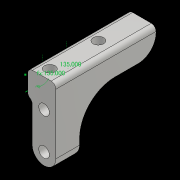
# Autodesk Inventor part: small_gpu_02
Saved by Autodesk Inventor 2018.2 (Build 222227000, 227)
## iProperties
Created: 2020-06-13
Part Number: small_gpu_02
Material: アルミニウム 6061
Document SubType Name: Modeling
Designer: gisen
Density: 2.7 g/cm^3
Appearance: アルミニウム - フラット
Author: gisen
## iProperties of the stored document small_gpu_02_3D プリント.ipt
Created: 2020-06-13
Part Number: small_gpu_02_3D プリント
Material: アルミニウム 6061
Document SubType Name: Modeling
Designer: gisen
Density: 2.7 g/cm^3
Appearance: アルミニウム - フラット
Author: gisen
Autodesk Inventor part; units mm, degrees
ref_plane "YZ Plane" through (0, 0, 0) normal (1, 0, 0) x (0, 1, 0)
ref_plane "XZ Plane" through (0, 0, 0) normal (0, 1, 0) x (-1, 0, 0)
ref_plane "XY Plane" through (0, 0, 0) normal (0, 0, 1) x (1, 0, 0)
sketch "スケッチ1" plane through (0, 0, 0) normal (0, 0, 1) x (1, 0, 0)
  line L0 (0, 0) -> (25.5, 0)
  line L1 (25.5, 0) -> (25.5, 41.76)
  line L2 (25.5, 41.76) -> (0, 41.76)
  line L3 (0, 41.76) -> (0, 0)
  line L4 (0, 3) -> (25.5, 3) construction
  line L5 (13.5, 41.76) -> (13.5, 0) construction
  line L6 (12, 41.76) -> (12, 0) construction
  line L7 (12, 7.267) -> (13.5, 7.267)
  line L8 (13.5, 7.267) -> (13.5, 17.554)
  line L9 (13.5, 17.554) -> (12, 17.554)
  line L10 (12, 17.554) -> (12, 7.267)
  line L11 (12, 27.612) -> (13.5, 27.612)
  line L12 (13.5, 27.612) -> (13.5, 37.899)
  line L13 (13.5, 37.899) -> (12, 37.899)
  line L14 (12, 37.899) -> (12, 27.612)
  dimension "d0" = 3
  dimension "d1" = 38.76
  dimension "d2" = 1.5
  dimension "d3" = 12
  dimension "d4" = 25.5
  dimension "d5" = 4.267
  dimension "d6" = 10.287
  dimension "d7" = 10.058
  dimension "d8" = 10.287
  dimension "d11" = 12
  constraints: 30 end point, 10 point on line, 7 parallel, 4 horizontal, 4 perpendicular
  measures "d0" distance between parallel lines of L0 L4
  measures "d1" distance between parallel lines of L4 L2
  measures "d2" distance between parallel lines of L5 L6
  measures "d3" distance between parallel lines of L1 L5
  measures "d4" distance between parallel lines of L1 L3
  measures "d5" distance between parallel lines of L4 L7
  measures "d6" distance between parallel lines of L9 L7
  measures "d7" distance between parallel lines of L9 L11
  measures "d8" distance between parallel lines of L13 L11
  measures "d11" distance between parallel lines of L3 L6
extrude "押し出し1" add sketch "スケッチ1" along normal mid plane 7.5
sketch "スケッチ2" plane through (0, 0, -3.75) normal (0, -1, 0) x (1, 0, 0)
  line L0 (25.5, 7.5) -> (0, 7.5) projected
  line L1 (0, 7.5) -> (25.5, 7.5)
  line L2 (25.5, 7.5) -> (25.5, 2.5)
  line L3 (25.5, -2.5) -> (20.5, -2.5)
  line L4 (0, -2.5) -> (0, 2.5)
  line L5 (25.5, 2.5) -> (0, 2.5) construction
  line L6 (0, 3.75) -> (0, 7.5) construction
  arc A0 (0, 2.5) -> (5, -2.5) centre (5, 2.5) ccw
  line L7 (5, 2.5) -> (5, -2.5) construction
  line L8 (5, 2.5) -> (0, 2.5) construction
  arc A1 (20.5, -2.5) -> (25.5, 2.5) centre (20.5, 2.5) ccw
  line L9 (20.5, 2.5) -> (20.5, -2.5) construction
  line L10 (20.5, 2.5) -> (25.5, 2.5) construction
  line L11 (25.5, 0) -> (25.5, 7.5) projected
  line L12 (0, 2.5) -> (0, 7.5)
  line L13 (5, -2.5) -> (0, -2.5)
  line L14 (20.5, -2.5) -> (5, -2.5)
  line L15 (25.5, 2.5) -> (25.5, -2.5)
  dimension "d12" = 90
  dimension "d13" = 90
  dimension "d14" = 10
  dimension "d15" = 5
  constraints: 26 end point, 7 parallel, 4 perpendicular, 4 point on circle, 4 point on line, 2 centre point, 1 horizontal
  measures "d12" angle of L8 L7
  measures "d13" angle of L9 L10
  measures "d14" distance between parallel lines of L13 L0
  measures "d15" distance between parallel lines of L5 L1
extrude "押し出し2" add sketch "スケッチ2" against normal up to surface (7.267 mm away)
extrude "押し出し3" [suppressed]
ref_plane "作業平面1" through (0, 0, -1.25) normal (0, 0, 1) x (1, 0, 0)
sketch "スケッチ3" plane through (0, 0, 3.75) normal (0, -1, 0) x (1, 0, 0)
  arc A0 (0, -5) -> (5, -10) centre (5, -5) ccw construction
  arc A1 (20.5, -10) -> (25.5, -5) centre (20.5, -5) ccw construction
  circle A2 centre (5, -5) radius 2.25
  circle A3 centre (20.5, -5) radius 2.25
  point P0 (0, -3.75)
  dimension "d20" = 4.5
  dimension "d21" = 4.5
  constraints: 2 centre point, 2 coincident
  measures "d20" diameter of A2
  measures "d21" diameter of A3
extrude "押し出し4" cut sketch "スケッチ3" against normal up to surface (41.76 mm away)
sketch "スケッチ4" plane through (0.6699, 41.76, -3.75) normal (0, 1, 0) x (1, 0, 0)
  circle A0 centre (19.8301, -2.5) radius 2.25 construction
  circle A1 centre (4.3301, -2.5) radius 2.25 construction
  line L0 (0, 0) -> (24.1603, 0) projected
  line L1 (19.8301, 0) -> (19.8301, -2.5) construction
  line L2 (17.5801, 0) -> (17.5801, -2.5)
  line L3 (22.0801, -2.5) -> (22.0801, 0)
  arc A2 (22.0801, 0) -> (17.5801, 0) centre (19.8301, 0) ccw
  arc A3 (17.5801, -2.5) -> (22.0801, -2.5) centre (19.8301, -2.5) ccw
  line L4 (4.3301, -0.25) -> (4.3301, -2.5) construction
  line L5 (2.0801, -0.25) -> (2.0801, -2.5)
  line L6 (6.5801, -2.5) -> (6.5801, -0.25)
  arc A4 (6.5801, -0.25) -> (2.0801, -0.25) centre (4.3301, -0.25) ccw
  arc A5 (2.0801, -2.5) -> (6.5801, -2.5) centre (4.3301, -2.5) ccw
  point P0 (-0.6699, -3.75)
  point P1 (19.8301, -1.25)
  point P2 (4.3301, -1.375)
  constraints: 16 end point, 8 point on circle, 8 tangent, 4 centre point, 3 parallel, 2 midpoint, 1 concentric, 1 perpendicular, 1 point on line, 1 vertical alignment, 2 other
extrude "押し出し5" [suppressed]
sketch "スケッチ5" plane through (12, 7.267, 3.75) normal (1, 0, 0) x (0, 0, -1)
  line L0 (0, 0) -> (7.5, 0) construction
  line L1 (7.5, 10.287) -> (0, 10.287) construction
  line L2 (7.5, 10.287) -> (10, 12.787)
  line L3 (10, 12.787) -> (10, -2.5)
  line L4 (10, -2.5) -> (7.5, 0)
  line L5 (7.5, 0) -> (7.5, 10.287)
  line L6 (10, -7.267) -> (10, 0) projected
  point P0 (3.75, -7.267)
  dimension "d28" = 135
  dimension "d29" = 135
  constraints: 9 end point, 2 vertical, 1 point on line
  measures "d28" angle of L5 L2
  measures "d29" angle of L4 L5
sketch "スケッチ6" plane through (0, 0, 3.75) normal (0, 0, 1) x (1, 0, 0)
  line L0 (12, 27.612) -> (12, 37.899) construction
  line L1 (12, 37.899) -> (13.5, 37.899) construction
  line L2 (13.5, 37.899) -> (13.5, 27.612) construction
  line L3 (13.5, 27.612) -> (12, 27.612) construction
  line L4 (12, 7.267) -> (12, 17.554) construction
  line L5 (12, 17.554) -> (13.5, 17.554) construction
  line L6 (13.5, 17.554) -> (13.5, 7.267) construction
  line L7 (13.5, 7.267) -> (12, 7.267) construction
  line L8 (0, 0) -> (25.5, 0) construction
  line L9 (25.5, 41.76) -> (0, 41.76) construction
  line L10 (13.625, 27.487) -> (13.625, 38.024)
  line L11 (13.625, 38.024) -> (11.875, 38.024)
  line L12 (11.875, 38.024) -> (11.875, 27.487)
  line L13 (11.875, 27.487) -> (13.625, 27.487)
  line L14 (13.625, 7.142) -> (13.625, 17.679)
  line L15 (13.625, 17.679) -> (11.875, 17.679)
  line L16 (11.875, 17.679) -> (11.875, 7.142)
  line L17 (11.875, 7.142) -> (13.625, 7.142)
  line L18 (0, 41.76) -> (0, 0) projected
  line L19 (25.5, 0) -> (25.5, 41.76) projected
  dimension "d32" = 0.125
  dimension "d33" = 0.125
  constraints: 16 end point, 6 other
  measures "d32" distance between parallel lines of L2 L10
  measures "d33" distance between parallel lines of L6 L14
extrude "押し出し7" cut sketch "スケッチ6" against normal through all
sketch "スケッチ8" plane through (0, 0, 3.75) normal (0, -1, 0) x (1, 0, 0)
  line L0 (13.625, 0) -> (13.625, -10) construction
  line L1 (0, 0) -> (0, -10) projected
  line L2 (0, 0) -> (13.625, 0)
  line L3 (13.625, 0) -> (13.625, -10)
  line L4 (13.625, -10) -> (0, -10)
  line L5 (0, -10) -> (0, 0)
  point P0 (0, -3.75)
  constraints: 8 end point, 2 parallel, 1 horizontal, 1 perpendicular
extrude "押し出し10" cut sketch "スケッチ8" against normal up to surface (41.76 mm away)
sketch "スケッチ9" plane through (25.5, 7.267, -3.75) normal (0, 1, 0) x (1, 0, 0)
  line L0 (-11.875, 2.5) -> (-11.875, 0) projected
  line L1 (0, 0) -> (-11.875, 0) projected
  line L2 (0, 0) -> (0, 2.5) projected
  line L3 (0, 2.5) -> (-11.875, 2.5) projected
  point P0 (-25.5, -3.75)
extrude "押し出し11" add sketch "スケッチ9" along normal up to surface (34.493 mm away)
sketch "スケッチ10" plane through (25.5, 0, -6.25) normal (0, -1, 0) x (1, 0, 0)
  line L0 (-11.875, 0) -> (0, 0) projected
  line L1 (-11.875, 0) -> (0, 0)
  line L2 (0, 0) -> (0, -22.5)
  line L3 (0, -22.5) -> (-11.875, -22.5)
  line L4 (-11.875, -22.5) -> (-11.875, 0)
  circle A0 centre (-5, 5) radius 2.25 construction
  line L5 (-5, 5) -> (-5, -17.5) construction
  circle A1 centre (-5, -17.5) radius 2.25
  point P0 (-25.5, 6.25)
  dimension "d46" = 22.5
  dimension "d47" = 5
  dimension "d48" = 5
  constraints: 10 end point, 2 parallel, 1 centre point, 1 coincident, 1 equal radius, 1 horizontal, 1 perpendicular, 1 vertical
  measures "d46" distance of L5.start L5.end
  measures "d47" distance between parallel lines of L5 L2
  measures "d48" distance from line of L3 L5.end
extrude "押し出し12" add sketch "スケッチ10" against normal up to surface (41.76 mm away)
sketch "スケッチ12" plane through (13.625, 0, 3.75) normal (0, -1, 0) x (1, 0, 0)
  circle A0 centre (6.875, -5) radius 2.25 projected
  point P0 (-13.625, -3.75)
extrude "押し出し14" add sketch "スケッチ12" against normal up to surface (41.76 mm away)
sketch "スケッチ11" plane through (0, 0, 3.75) normal (0, 0, 1) x (1, 0, 0)
  line L0 (22.75, 0) -> (18.25, 0) construction
  line L1 (18.723, 0) -> (18.723, 3.589) construction
  circle A0 centre (18.723, 3.589) radius 2.25
  line L2 (13.625, 41.76) -> (13.625, 0) projected
  line L3 (18.723, 3.589) -> (18.723, 24.163) construction
  line L4 (18.25, 0) -> (18.25, 41.76) construction
  circle A1 centre (18.723, 24.163) radius 2.25
  point P0 (0, 0)
  dimension "d51" = 4.5
  dimension "d52" = 3.589
  dimension "d53" = 5.098
  dimension "d54" = 20.574
  constraints: 4 end point, 2 centre point, 2 coincident, 1 equal radius, 1 parallel, 1 point on line, 1 vertical
  measures "d51" diameter of A0
  measures "d52" distance of L1.start L1.end
  measures "d53" distance between parallel lines of L2 L1
  measures "d54" distance of L3.start L3.end
extrude "押し出し13" cut sketch "スケッチ11" against normal blind 7.5
sketch "スケッチ13" plane through (13.625, 0, 3.75) normal (0, -1, 0) x (1, 0, 0)
  circle A0 centre (6.875, -27.5) radius 2.25 construction
  line L0 (6.875, -27.5) -> (6.875, -12) construction
  circle A1 centre (6.875, -12) radius 2.25
  point P0 (-13.625, -3.75)
  dimension "d59" = 15.5
  constraints: 2 end point, 1 centre point, 1 coincident, 1 equal radius, 1 vertical
  measures "d59" distance of L0.start L0.end
extrude "押し出し15" cut sketch "スケッチ13" against normal up to surface (41.76 mm away)
sketch "スケッチ14" plane through (13.625, 0, 3.75) normal (0, -1, 0) x (1, 0, 0)
  line L0 (2.848, -7.5) -> (7.348, -7.5) construction
  line L1 (2.848, 0) -> (7.348, 0) construction
  line L2 (0, -32.5) -> (0, 0) projected
  line L3 (0, -32.5) -> (1.875, -32.5)
  line L4 (1.875, -32.5) -> (1.875, -10.5)
  line L5 (1.875, -10.5) -> (0, -10.5)
  line L6 (0, -10.5) -> (0, -32.5)
  circle A0 centre (6.875, -27.5) radius 2.25 projected
  point P0 (-13.625, -3.75)
  dimension "d62" = 3
  dimension "d63" = 5
  constraints: 8 end point, 2 parallel, 1 horizontal, 1 perpendicular
  measures "d62" distance between parallel lines of L5 L0
  measures "d63" distance from line of A0.centre L4
extrude "押し出し16" cut sketch "スケッチ14" against normal up to surface (41.76 mm away) contours L2 L5 L4 L3
fillet "フィレット4" radius 2 1 edges at (15.5, 20.88, -6.75)
fillet "フィレット5" radius 5 2 edges at (25.5, 20.88, -28.75) (15.5, 20.88, -28.75)
sketch "スケッチ16" plane through (13.625, 41.76, 3.75) normal (0, 1, 0) x (1, 0, 0)
  arc A0 (11.875, 27.5) -> (1.875, 27.5) centre (6.875, 27.5) ccw projected
  line L0 (1.875, 27.5) -> (1.875, 12.4961) projected
  arc A1 (0, 10.5) -> (1.875, 12.4961) centre (-0.125, 12.4961) ccw projected
  line L1 (0, 10.5) -> (0, 0) projected
  line L2 (11.875, 0) -> (0, 0) projected
  line L3 (11.875, 27.5) -> (11.875, 0) projected
  circle A2 centre (6.875, 27.5) radius 2.25 projected
  circle A3 centre (6.875, 12) radius 2.25 projected
  point P0 (-13.625, 3.75)
extrude "押し出し17" add sketch "スケッチ16" along normal blind 7.928
sketch "スケッチ17" plane through (0, 0, 3.75) normal (0, 0, 1) x (1, 0, 0)
  circle A0 centre (18.723, 3.589) radius 2.25 construction
  circle A1 centre (18.723, 24.163) radius 2.25 construction
  line L0 (18.723, 3.589) -> (18.723, 24.163) construction
  line L1 (18.25, 0) -> (18.25, 49.688) construction
  line L2 (18.723, 24.163) -> (18.723, 44.737) construction
  line L3 (18.723, 44.737) -> (18.723, 65.311) construction
  circle A2 centre (18.723, 44.737) radius 2.25
  circle A3 centre (18.723, 65.311) radius 2.25
  point P0 (0, 0)
  constraints: 6 end point, 2 centre point, 2 coincident, 2 collinear, 2 equal radius, 2 point on line, 1 parallel
extrude "押し出し18" cut sketch "スケッチ17" against normal blind 7.5
fillet "フィレット6" radius 2 1 edges at (13.625, 20.88, -6.7539)
fillet "フィレット7" radius 2 2 edges at (13.625, 24.844, 3.75) (25.5, 24.844, 3.75)
sketch "スケッチ18" plane through (25.5, 0, -23.75) normal (1, 0, 0) x (0, 0, -1)
  line L0 (-27.5, 49.688) -> (-27.5, 0) projected
  line L1 (-27.5, 41.76) -> (-7.75, 41.76)
  line L2 (0, 0) -> (-25.5, 0) projected
  arc A0 (5, 29.01) -> (-7.75, 41.76) centre (-7.75, 29.01) ccw
  line L3 (-7.75, 29.01) -> (5, 29.01) construction
  line L4 (-7.75, 29.01) -> (-7.75, 41.76) construction
  line L5 (-27.5, 41.76) -> (-27.5, 50.688)
  line L6 (-27.5, 50.688) -> (6, 50.688)
  line L7 (6, 50.688) -> (6, 29.01)
  line L8 (6, 29.01) -> (5, 29.01)
  line L9 (-25.5, 49.688) -> (0, 49.688) projected
  line L10 (5, 0) -> (5, 49.688) construction
  point P0 (-23.75, 0)
  dimension "d75" = 41.76
  dimension "d76" = 90
  dimension "d77" = 12.75
  dimension "d78" = 1
  dimension "d79" = 6
  constraints: 14 end point, 3 perpendicular, 3 point on line, 2 point on circle, 1 centre point, 1 horizontal, 1 vertical
  measures "d75" distance between parallel lines of L2 L1
  measures "d76" angle of L3 L4
  measures "d77" radius of A0
  measures "d78" distance between parallel lines of L6 L9
  measures "d79" distance from line of L7 L2.start
extrude "押し出し19" cut sketch "スケッチ18" against normal up to surface (11.875 mm away)
sketch "スケッチ19" plane through (20.5, 0, -23.75) normal (0, -1, 0) x (1, 0, 0)
  arc A0 (5, 25.5) -> (3, 27.5) centre (3, 25.5) ccw projected
  line L0 (-4.875, 27.5) -> (3, 27.5) projected
  arc A1 (-4.875, 27.5) -> (-6.875, 25.5) centre (-4.875, 25.5) ccw projected
  line L1 (-6.875, 18.3928) -> (-6.875, 25.5) projected
  arc A2 (-6.875, 18.3928) -> (-5.9375, 16.6983) centre (-4.875, 18.3928) ccw projected
  arc A3 (-5, 15.0039) -> (-5.9375, 16.6983) centre (-7, 15.0039) ccw projected
  line L2 (-5, 15.0039) -> (-5, 0) projected
  arc A4 (-5, 0) -> (5, 0) centre (0, 0) ccw projected
  line L3 (5, 0) -> (5, 25.5) projected
  circle A5 centre (0, 0) radius 2.25 projected
  circle A6 centre (0, 15.5) radius 2.25 projected
  point P0 (-20.5, 23.75)
extrude "押し出し20" add sketch "スケッチ19" along normal blind 0.6
sketch "スケッチ20" plane through (25.5, 41.76, 1.75) normal (1, 0, 0) x (0, 0, -1)
  line L0 (8, 0) -> (30.5, 0)
  line L1 (30.5, 0) -> (30.5, -32.36)
  line L2 (30.5, -32.36) -> (23, -32.36)
  line L3 (8, 0) -> (8, -17.36)
  line L4 (7.1072, 0) -> (7.1072, -42.36) projected
  arc A0 (8, -17.36) -> (23, -32.36) centre (23, -17.36) ccw
  line L5 (-2, 0) -> (-2, -42.36) projected
  line L6 (25.5, -42.36) -> (30.5, -42.36) projected
  line L7 (30.5, -42.36) -> (30.5, -12.75) construction
  line L8 (17.75, 0) -> (0, 0) construction
  point P0 (1.75, -41.76)
  dimension "d84" = 10
  dimension "d85" = 10
  dimension "d86" = 15
  constraints: 8 end point, 2 perpendicular, 2 point on circle, 2 point on line, 2 tangent, 1 centre point, 1 horizontal, 1 parallel
  measures "d84" distance between parallel lines of L5 L3
  measures "d85" distance between parallel lines of L6 L2
  measures "d86" radius of A0
extrude "押し出し21" cut sketch "スケッチ20" against normal up to surface (11.875 mm away)
fillet "フィレット8" radius 7.5 1 edges at (16.6513, 41.76, -6.25)
equation "\"d8\" = d6"
equation "\"d11\" = d3"
equation "\"d29\" = d28"
equation "\"d33\" = d32"
equation "\"d48\" = d47"
